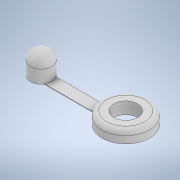
# Autodesk Inventor part: pipe form
Saved by Autodesk Inventor 2022 (Build 260153000, 153)
## iProperties
Created: 2022-06-06
Part Number: pipe form
Material: Generic
Document SubType Name: Modeling
Designer: dech3
Density: 1 g/cm^3
Appearance: Default
Author: dech3
Autodesk Inventor part; units mm, degrees
ref_plane "YZ Plane" through (0, 0, 0) normal (1, 0, 0) x (0, 1, 0)
ref_plane "XZ Plane" through (0, 0, 0) normal (0, 1, 0) x (-1, 0, 0)
ref_plane "XY Plane" through (0, 0, 0) normal (0, 0, 1) x (1, 0, 0)
sketch "Sketch1" plane through (0, 0, 0) normal (0, 1, 0) x (-1, 0, 0)
  circle A0 centre (0, 0) radius 4.5
  dimension "d0" = 9
  constraints: 2 coincident, 1 centre point
  measures "d0" diameter of A0
extrude "Extrusion1" add sketch "Sketch1" along normal blind 10
fillet "Fillet1" radius 4.5 1 edges at (4.5, 10, 0)
sketch "Sketch2" plane through (0, 0, 0) normal (0, -1, 0) x (1, 0, 0)
  line L0 (0, 2.5) -> (30, 2.5)
  line L1 (30, 2.5) -> (30, -2.5)
  line L2 (30, -2.5) -> (0, -2.5)
  line L3 (0, -2.5) -> (0, 2.5)
  point P0 (0, 0)
  dimension "d4" = 30
  dimension "d5" = 5
  dimension "d6" = 2.5
  constraints: 8 end point, 2 parallel, 1 horizontal, 1 perpendicular, 1 vertical alignment
  measures "d4" distance between parallel lines of L1 L3
  measures "d5" distance between parallel lines of L2 L0
  measures "d6" distance from line of L0 point (0, 0)
extrude "Extrusion2" add sketch "Sketch2" against normal blind 0.2
sketch "Sketch3" plane through (0, 0, 0) normal (0, -1, 0) x (1, 0, 0)
  line L0 (30, 2.5) -> (3.7417, 2.5) projected
  circle A0 centre (35.5, 0) radius 10
  circle A1 centre (0, 0) radius 0.101 projected
  circle A2 centre (35.5, 0) radius 5
  line L1 (30, 2.5) -> (30, -2.5) projected
  point P0 (4.3301, 2.5)
  dimension "d20" = 10
  dimension "d21" = 5
  dimension "d22" = 5.5
  constraints: 2 centre point, 1 concentric, 1 horizontal alignment
  measures "d20" diameter of A2
  measures "d21" radial gap between concentric circles of A0 A2
  measures "d22" distance from line of L1 A2.centre
extrude "Extrusion3" add sketch "Sketch3" against normal blind 5 contours A0
fillet "Fillet2" radius 2 4 edges at (25.5, 5, 0) (25.5, 0.2, 0) (25.8175, 0.1, -2.5) (25.8175, 0.1, 2.5)
body "Solid1"
